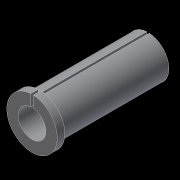
# Autodesk Inventor part: 迫緊環
Saved by Autodesk Inventor 2016 (Build 200138000, 138)
## iProperties
Created: 2016-02-22
Part Number: 迫緊環
Material: 一般
Document SubType Name: Modeling
Designer: ERIC
Density: 1 g/cm^3
Appearance: 預設
Author: ERIC
Autodesk Inventor part; units mm, degrees
ref_plane "YZ Plane" through (0, 0, 0) normal (1, 0, 0) x (0, 1, 0)
ref_plane "XZ Plane" through (0, 0, 0) normal (0, 1, 0) x (-1, 0, 0)
ref_plane "XY Plane" through (0, 0, 0) normal (0, 0, 1) x (1, 0, 0)
sketch "草圖1" plane through (0, 0, 0) normal (0, 1, 0) x (-1, 0, 0)
  circle A0 centre (0, 0) radius 10
  dimension "d0" = 20
  constraints: 1 centre point, 1 coincident
  measures "d0" diameter of A0
extrude "擠出1" add sketch "草圖1" along normal blind 3
sketch "草圖2" plane through (0, 3, 0) normal (0, 1, 0) x (1, 0, 0)
  circle A0 centre (0, 0) radius 8.3
  circle A1 centre (0, 0) radius 5.5
  dimension "d3" = 16.6
  dimension "d4" = 11
  constraints: 2 centre point, 2 coincident
  measures "d3" diameter of A0
  measures "d4" diameter of A1
extrude "擠出2" add sketch "草圖2" along normal blind 43 contours A0 | A1
sketch "草圖3" plane through (0, 0, 0) normal (0, -1, 0) x (1, 0, 0)
  circle A0 centre (0, 0) radius 5.5
  circle A1 centre (0, 0) radius 10 projected
  dimension "d19" = 11
  constraints: 1 centre point, 1 concentric
  measures "d19" diameter of A0
extrude "擠出3" cut sketch "草圖3" against normal blind 43 contours A0
sketch "草圖4" plane through (0, 46, 0) normal (0, 1, 0) x (1, 0, 0)
  point P0 (0, 0)
hole "孔1" at (0, 46, 0) direction (0, -1, 0) diameter 10 end through all
sketch "草圖5" plane through (0, 0, 0) normal (0, -1, 0) x (1, 0, 0)
  circle A0 centre (0, 0) radius 5 projected
  circle A1 centre (0, 0) radius 10 projected
  line L0 (0, 0) -> (0, 9.3404) construction
  line L1 (-0.5, 4.9749) -> (-0.5, 9.9875)
  line L2 (0.5, 4.9749) -> (0.5, 9.9875)
  dimension "d16" = 1
  constraints: 6 end point, 4 point on circle, 3 vertical, 1 other
  measures "d16" distance between parallel lines of L2 L1
extrude "擠出4" cut sketch "草圖5" against normal through all contours A0 L1 A1 L2 picked at (0.0556, 6.6643)
